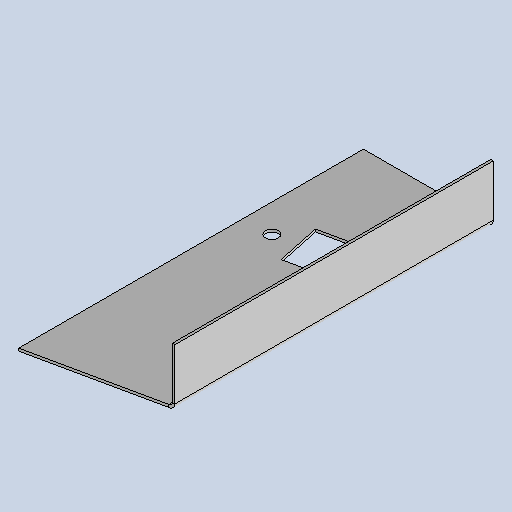
# Autodesk Inventor part: MNT-CDF-613 big way
Saved by Autodesk Inventor 2025 (Build 290162010, 162A)
## iProperties
Created: 2025-01-16
Part Number: MNT-CDF-613 big way
Material: Stainless Steel
Document SubType Name: Sheet Metal
Designer: user
Density: 8 g/cm^3
Flat Pattern Width: 14.3202 cm
Flat Pattern Length: 27.0671 cm
Flat Pattern Area: 387.606 cm^2
Sheet Metal Rule: AISI304 2mm Die16
Sheet Metal Width: 143.202 mm
Sheet Metal Length: 270.671 mm
Sheet Metal Area: 38760.644 mm^2
Appearance: Default
Author: pokla
Autodesk Inventor part; units mm, degrees
ref_plane "YZ Plane" through (0, 0, 0) normal (1, 0, 0) x (0, 1, 0)
ref_plane "XZ Plane" through (0, 0, 0) normal (0, 1, 0) x (-1, 0, 0)
ref_plane "XY Plane" through (0, 0, 0) normal (0, 0, 1) x (1, 0, 0)
sketch "Sketch1" plane through (0, 0, 0) normal (0, 0, 1) x (1, 0, 0)
  line L0 (-51, 125) -> (51, 125)
  line L1 (51, 125) -> (51, -125)
  line L2 (51, -125) -> (-51, -125)
  line L3 (-51, -125) -> (-51, 125)
  line L4 (-51, 125) -> (51, -125) construction
  point P0 (0, 0)
  point P1 (0, 0)
  dimension "d0" = 102
  dimension "d1" = 250
  measures "d0" distance of L0.start L0.end
  measures "d1" distance of L2.end L0.start
extrude "Plate1" add sketch "Sketch1" along normal blind 2
sketch "Sketch4" plane through (49, 125, 0) normal (1, 0, 0) x (0, 1, 0)
  line L0 (-250, 0) -> (0, 0)
  line L1 (0, 0) -> (0, 45)
  line L2 (0, 45) -> (-250, 45)
  line L3 (-250, 45) -> (-250, 0)
  constraints: 6 end point, 1 horizontal, 1 perpendicular, 1 vertical
edge flange "Flange1" height 45 angle 90 thickness 2 bend radius 2.75 thickness toward (1, 0, 0) relief round relief width 2 relief depth 1 edges at (51, 0, 2) wall of the first edge with corners at (49, -125, 0) (49, 125, 0) (49, 125, 45) (49, -125, 45)
bend "Bend1"
corner "Corner1"
sketch "Sketch5" plane through (0, 0, 0) normal (0, 0, -1) x (-1, 0, 0)
  line L0 (-46.25, 125) -> (-46.25, -125) projected
  line L1 (51, -125) -> (-46.25, -125) projected
  line L2 (51, 125) -> (51, -125) projected
  line L3 (-46.25, 125) -> (51, 125) projected
  line L4 (51, -125) -> (51, -145.6711)
  line L5 (-46.25, -125) -> (51, -125) projected
  line L6 (51, -145.6711) -> (-46.25, -125)
  point P0 (0, 0)
  dimension "d25" = 12
  constraints: 4 end point, 1 vertical
  measures "d25" angle of L1 L6
extrude "Extrusion2" add sketch "Sketch5" against normal up to surface (2 mm away) contours L1 L4 L6
sketch "Sketch7" plane through (0, 0, 0) normal (0, 0, 1) x (1, 0, 0)
  line L0 (46.25, -125) -> (-51, -145.6711) projected
  circle A0 centre (36.9805, 9.3484) radius 5.05
  line L1 (36.9805, 9.3484) -> (22.4267, 77.8187) construction
  line L2 (26.006, 24.9066) -> (18.7291, 59.1418)
  circle A1 centre (22.4267, 77.8187) radius 5.05
  line L3 (-28.9852, 31.1089) -> (36.9805, 9.3484) construction
  line L4 (26.006, 24.9066) -> (-15.5061, 51.8649) construction
  line L5 (18.7291, 59.1418) -> (-15.5061, 51.8649)
  line L6 (-8.2292, 17.6297) -> (26.006, 24.9066)
  line L7 (18.7291, 59.1418) -> (-8.2292, 17.6297) construction
  line L8 (-15.5061, 51.8649) -> (-8.2292, 17.6297)
  line L9 (22.3675, 42.0242) -> (-28.9852, 31.1089) construction
  line L10 (22.4267, 77.8187) -> (-28.9852, 31.1089) construction
  circle A2 centre (-28.9852, 31.1089) radius 5.05
  point P0 (0, 0)
  point P1 (-47.5274, -178.5141)
  point P2 (5.2499, 38.3858)
  point P3 (-51, -145.6711)
  dimension "d32" = 35
  dimension "d33" = 35
  dimension "d34" = 10.1
  dimension "d35" = 70
  dimension "d36" = 60
  dimension "d37" = 25
  constraints: 20 end point, 3 centre point, 3 midpoint, 3 parallel, 1 equal radius, 1 perpendicular, 4 other
  measures "d32" distance of L6.start L4.end
  measures "d33" distance of L4.end L2.end
  measures "d34" diameter of A2
  measures "d35" distance of L1.start L1.end
  measures "d36" distance from line of L3.start L1
  measures "d37" distance from line of L1 point (5.25, 38.386)
extrude "Extrusion3" cut sketch "Sketch7" along normal through all
equation "\"d33\" = d32"
equation "\"d2\" = Thickness"
equation "\"d15\" = BendReliefWidth"
equation "\"d16\" = BendReliefDepth"
equation "\"d17\" = MinimumRemnant"
equation "\"d18\" = TransitionRadius"
equation "\"d21\" = BendRadius"
equation "\"d22\" = CornerReliefSize"
equation "\"d23\" = GapSize"
equation "\"d24\" = JacobiRadiusSize"
equation "\"BendReliefWidth\" = Thickness"
equation "\"BendReliefDepth\" = 0.5 * Thickness"
equation "\"CornerReliefSize\" = 4 * Thickness"
equation "\"MinimumRemnant\" = 2 * Thickness"
equation "\"TransitionRadius\" = BendRadius"
equation "\"JacobiRadiusSize\" = BendRadius"
equation "\"GapSize\" = Thickness"
equation "\"Thickness\" = 2"
equation "\"BendRadius\" = 2.75"
body "Solid1"
